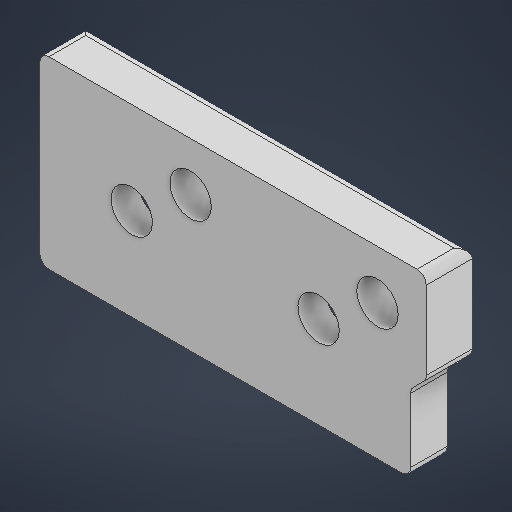
# Autodesk Inventor part: gpu_hold_plate
Saved by Autodesk Inventor 2026.2 (Build 302298010, 298A)
## iProperties
Created: 2025-02-02
Part Number: gpu_hold_plate
Material: 一般
Document SubType Name: Modeling
Designer: nyxeon
Density: 1 g/cm^3
Appearance: 既定
Author: nyxeon
Autodesk Inventor part; units mm, degrees
ref_plane "YZ Plane" through (0, 0, 0) normal (1, 0, 0) x (0, 1, 0)
ref_plane "XZ Plane" through (0, 0, 0) normal (0, 1, 0) x (-1, 0, 0)
ref_plane "XY Plane" through (0, 0, 0) normal (0, 0, 1) x (1, 0, 0)
sketch "スケッチ1" plane through (0, 0, 0) normal (0, 0, 1) x (1, 0, 0)
  arc A0 (-17.9, -5.9192) -> (-17.6, -6.2192) centre (-17.6, -5.9192) ccw construction
  line L0 (-17.6, -6.2192) -> (-11.8244, -6.2192) construction
  line L1 (-11.8244, -6.2192) -> (-9.5, -2.219) projected
  arc A1 (-9.2172, -2.0192) -> (-9.5, -2.219) centre (-9.2172, -2.3192) ccw projected
  line L2 (-9.2172, -2.0192) -> (-6.9328, -2.0192) projected
  arc A2 (-6.65, -2.219) -> (-6.9328, -2.0192) centre (-6.9328, -2.3192) ccw projected
  line L3 (-6.65, -2.219) -> (-4.3256, -6.2192) projected
  line L4 (-4.3256, -6.2192) -> (8.4756, -6.2192) construction
  line L5 (8.4756, -6.2192) -> (10.8, -2.219) projected
  arc A3 (11.0828, -2.0192) -> (10.8, -2.219) centre (11.0828, -2.3192) ccw projected
  line L6 (11.0828, -2.0192) -> (13.3672, -2.0192) projected
  arc A4 (13.65, -2.219) -> (13.3672, -2.0192) centre (13.3672, -2.3192) ccw projected
  line L7 (13.65, -2.219) -> (15.9744, -6.2192) projected
  line L8 (15.9744, -6.2192) -> (21.25, -6.2192) construction
  arc A5 (21.25, -6.2192) -> (21.55, -5.9192) centre (21.25, -5.9192) ccw construction
  line L9 (21.55, -2.3692) -> (21.55, -5.9192) construction
  arc A6 (21.55, -2.3692) -> (21.25, -2.0692) centre (21.25, -2.3692) ccw construction
  line L10 (21.25, -2.0692) -> (17.65, -2.0692) construction
  arc A7 (17.65, 2.2308) -> (17.65, -2.0692) centre (17.65, 0.0808) ccw construction
  line L11 (17.65, 2.2308) -> (21.25, 2.2308) construction
  arc A8 (21.25, 2.2308) -> (21.55, 2.5308) centre (21.25, 2.5308) ccw construction
  line L12 (21.55, 4.8808) -> (21.55, 2.5308) construction
  line L13 (21.55, 4.8808) -> (-17.9, 4.8808) construction
  line L14 (-17.9, 4.8808) -> (-17.9, -5.9192) construction
  line L15 (1.3, 1.9308) -> (1.3, -1.7692) construction
  arc A9 (1, -2.0692) -> (1.3, -1.7692) centre (1, -1.7692) ccw construction
  line L16 (1, -2.0692) -> (-2.5, -2.0692) construction
  arc A10 (-2.5, 2.2308) -> (-2.5, -2.0692) centre (-2.5, 0.0808) ccw construction
  line L17 (-2.5, 2.2308) -> (1, 2.2308) construction
  arc A11 (1.3, 1.9308) -> (1, 2.2308) centre (1, 1.9308) ccw construction
  line L18 (-17.9, 5.3808) -> (21.55, 5.3808) construction
  circle A12 centre (-0.85, 0.0808) radius 2.15 construction
  line L19 (-0.85, 0.0808) -> (-2.5, 0.0808) construction
  circle A13 centre (-1.675, 0.0808) radius 2.25
  line L20 (64.025, 2.5048) -> (64.025, 91.3712) construction
  line L21 (-65.975, 91.3712) -> (-65.975, 2.5048) construction
  line L22 (64.025, 5.3808) -> (-65.975, 5.3808)
  circle A14 centre (18.625, 0.0808) radius 2.25
  circle A15 centre (38.925, 0.0808) radius 2.25
  circle A16 centre (59.225, 0.0808) radius 2.25
  circle A17 centre (-21.975, 0.0808) radius 2.25
  circle A18 centre (-1.675, 0.0808) radius 2.25
  circle A19 centre (18.625, 0.0808) radius 2.25
  circle A20 centre (38.925, 0.0808) radius 2.25
  circle A21 centre (-42.275, 0.0808) radius 2.25
  circle A22 centre (-21.975, 0.0808) radius 2.25
  circle A23 centre (-1.675, 0.0808) radius 2.25
  circle A24 centre (18.625, 0.0808) radius 2.25
  circle A25 centre (-62.575, 0.0808) radius 2.25
  circle A26 centre (-42.275, 0.0808) radius 2.25
  circle A27 centre (-21.975, 0.0808) radius 2.25
  circle A28 centre (-1.675, 0.0808) radius 2.25
  line L23 (64.025, 5.3808) -> (64.025, -6.2192)
  line L24 (64.025, -6.2192) -> (-65.975, -6.2192)
  line L25 (-65.975, -6.2192) -> (-65.975, 5.3808)
  point P0 (0, 0)
  dimension "d1" = 4.5
  dimension "d4" = 20.3
  dimension "d7" = 20.3
  constraints: 17 centre point, 10 end point, 5 point on line, 4 horizontal, 3 tangent, 1 collinear, 1 midpoint, 1 perpendicular, 30 other
  measures "d1" diameter of A13
  measures "d4" distance of A13.centre A14.centre
  measures "d7" distance of A13.centre A17.centre
extrude "押し出し1" add sketch "スケッチ1" along normal blind 5 contours L24 L25 L22 L23 L7 A4 L6 A3 L5 L3 A2 L2 A1 L1 | L1 A1 L2 A2 L3 L24 | L5 A3 L6 A4 L7 L24 | A16 | A25
sketch "スケッチ3" plane through (0, 0, 0) normal (0, 0, -1) x (-1, 0, 0)
  line L0 (9.5, -2.219) -> (11.8244, -6.2192) projected
  arc A0 (9.5, -2.219) -> (9.2172, -2.0192) centre (9.2172, -2.3192) ccw projected
  line L1 (6.9328, -2.0192) -> (9.2172, -2.0192) projected
  arc A1 (6.9328, -2.0192) -> (6.65, -2.219) centre (6.9328, -2.3192) ccw projected
  line L2 (4.3256, -6.2192) -> (6.65, -2.219) projected
  line L3 (65.975, -6.2192) -> (-64.025, -6.2192) projected
  point P0 (0, 0)
extrude "押し出し2" cut sketch "スケッチ3" against normal through all
pattern_linear "矩形状パターン1" count 4 spacing 20.3 along (1, 0, 0) count 3 spacing 20.3 along (-1, 0, 0) of "押し出し2"
fillet "フィレット1" radius 1 1 edges at (-0.975, 5.3808, 0)
sketch "スケッチ7" plane through (0, 0, 5) normal (0, 0, 1) x (1, 0, 0)
  line L0 (-52.4244, -6.2192) -> (-50.1, -2.219) projected
  arc A0 (-49.8172, -2.0192) -> (-50.1, -2.219) centre (-49.8172, -2.3192) ccw projected
  line L1 (-49.8172, -2.0192) -> (-47.5328, -2.0192) projected
  arc A1 (-47.25, -2.219) -> (-47.5328, -2.0192) centre (-47.5328, -2.3192) ccw projected
  line L2 (-47.25, -2.219) -> (-44.9256, -6.2192) projected
  line L3 (-32.1244, -6.2192) -> (-29.8, -2.219) projected
  arc A2 (-29.5172, -2.0192) -> (-29.8, -2.219) centre (-29.5172, -2.3192) ccw projected
  line L4 (-29.5172, -2.0192) -> (-27.2328, -2.0192) projected
  arc A3 (-26.95, -2.219) -> (-27.2328, -2.0192) centre (-27.2328, -2.3192) ccw projected
  line L5 (-26.95, -2.219) -> (-24.6256, -6.2192) projected
  line L6 (-11.8244, -6.2192) -> (-9.5, -2.219) projected
  arc A4 (-9.2172, -2.0192) -> (-9.5, -2.219) centre (-9.2172, -2.3192) ccw projected
  line L7 (-9.2172, -2.0192) -> (-6.9328, -2.0192) projected
  arc A5 (-6.65, -2.219) -> (-6.9328, -2.0192) centre (-6.9328, -2.3192) ccw projected
  line L8 (-6.65, -2.219) -> (-4.3256, -6.2192) projected
  line L9 (8.4756, -6.2192) -> (10.8, -2.219) projected
  arc A6 (11.0828, -2.0192) -> (10.8, -2.219) centre (11.0828, -2.3192) ccw projected
  line L10 (11.0828, -2.0192) -> (13.3672, -2.0192) projected
  arc A7 (13.65, -2.219) -> (13.3672, -2.0192) centre (13.3672, -2.3192) ccw projected
  line L11 (13.65, -2.219) -> (15.9744, -6.2192) projected
  line L12 (28.7756, -6.2192) -> (31.1, -2.219) projected
  arc A8 (31.3828, -2.0192) -> (31.1, -2.219) centre (31.3828, -2.3192) ccw projected
  line L13 (31.3828, -2.0192) -> (33.6672, -2.0192) projected
  arc A9 (33.95, -2.219) -> (33.6672, -2.0192) centre (33.6672, -2.3192) ccw projected
  line L14 (33.95, -2.219) -> (36.2744, -6.2192) projected
  line L15 (49.0756, -6.2192) -> (51.4, -2.219) projected
  arc A10 (51.6828, -2.0192) -> (51.4, -2.219) centre (51.6828, -2.3192) ccw projected
  line L16 (51.6828, -2.0192) -> (53.9672, -2.0192) projected
  arc A11 (54.25, -2.219) -> (53.9672, -2.0192) centre (53.9672, -2.3192) ccw projected
  line L17 (54.25, -2.219) -> (56.5744, -6.2192) projected
  line L18 (-52.4244, -6.2192) -> (-44.9256, -6.2192)
  line L19 (-24.6256, -6.2192) -> (-26.95, -2.219) projected
  line L20 (-32.1244, -6.2192) -> (-24.6256, -6.2192)
  line L21 (-9.5, -2.219) -> (-11.8244, -6.2192) projected
  line L22 (-11.8244, -6.2192) -> (-4.3256, -6.2192)
  line L23 (15.9744, -6.2192) -> (8.4756, -6.2192)
  line L24 (36.2744, -6.2192) -> (33.95, -2.219) projected
  line L25 (28.7756, -6.2192) -> (36.2744, -6.2192)
  line L26 (49.0756, -6.2192) -> (56.5744, -6.2192)
  point P0 (0, 0)
  constraints: 12 end point, 4 horizontal
extrude "押し出し5" add sketch "スケッチ7" against normal blind 4
sketch "スケッチ8" plane through (0, 0, 5) normal (0, 0, 1) x (1, 0, 0)
  circle A0 centre (-42.275, 0.0808) radius 2.25 projected
  circle A1 centre (-21.975, 0.0808) radius 2.25 projected
  line L0 (-42.275, 0.0808) -> (-21.975, 0.0808) construction
  line L1 (-21.975, 0.0808) -> (-32.125, 0.0808) construction
  line L2 (-48.675, -4.6192) -> (-28.375, -4.6192) construction
  circle A2 centre (-48.675, -4.6192) radius 2.25
  circle A3 centre (-28.375, -4.6192) radius 2.25
  line L3 (-65.975, -6.2192) -> (64.025, -6.2192) projected
  line L4 (-58.675, -6.2192) -> (-18.375, -6.2192)
  line L5 (-18.375, -6.2192) -> (-18.375, -14.6192)
  line L6 (-18.375, -14.6192) -> (-58.675, -14.6192)
  line L7 (-58.675, -14.6192) -> (-58.675, -6.2192)
  line L8 (-65.975, 5.3808) -> (64.025, 5.3808) projected
  line L9 (-27.2328, -2.0192) -> (-29.5172, -2.0192) construction
  point P0 (0, 0)
  point P1 (-38.525, -14.6192)
  point P2 (-18.375, -6.2192)
  point P3 (-38.525, -4.6192)
  point P4 (-28.375, -2.0192)
  point P5 (-28.375, -2.0192)
  dimension "d43" = 20.3
  dimension "d44" = 4.5
  dimension "d45" = 10
  dimension "d46" = 10
  dimension "d53" = 6.4
  dimension "d54" = 10
  dimension "d62" = 4.5
  dimension "d63" = 20.3
  constraints: 14 end point, 5 midpoint, 3 coincident, 3 horizontal, 2 centre point, 2 parallel, 2 vertical alignment, 1 equal radius, 1 perpendicular, 1 point on line
  measures "d43" distance of L2.start L2.end
  measures "d44" diameter of A2
  measures "d45" distance from line of L6 L2.end
  measures "d46" distance from line of L2.start L7
  measures "d53" horizontal distance of point (-38.525, -4.619) L1.end
  measures "d54" distance between parallel lines of L2 L8
  measures "d62" diameter of A0
  measures "d63" distance of L0.start L0.end
extrude "押し出し6" add sketch "スケッチ8" against normal up to surface (4 mm away) contours A2 L3 A3 L5 L6 L7
sketch "スケッチ10" plane through (0, 0, 5) normal (0, 0, 1) x (1, 0, 0)
  arc A0 (-50.2569, -6.2192) -> (-47.0931, -6.2192) centre (-48.675, -4.6192) ccw construction
  arc A1 (-29.9569, -6.2192) -> (-26.7931, -6.2192) centre (-28.375, -4.6192) ccw construction
  circle A2 centre (-48.675, -4.6192) radius 2.25
  circle A3 centre (-28.375, -4.6192) radius 2.25
  point P0 (0, 0)
  constraints: 2 centre point, 2 coincident
extrude "押し出し8" cut sketch "スケッチ10" against normal through all
sketch "スケッチ11" plane through (0, 0, 1) normal (0, 0, -1) x (-1, 0, 0)
  circle A0 centre (28.375, -4.6192) radius 2.25 construction
  circle A1 centre (48.675, -4.6192) radius 2.25 construction
  circle A2 centre (28.375, -4.6192) radius 4.15
  circle A3 centre (48.675, -4.6192) radius 4.15
  point P0 (0, 0)
  dimension "d57" = 8.3
  constraints: 2 centre point, 2 coincident, 1 equal radius
  measures "d57" diameter of A2
extrude "押し出し9" cut sketch "スケッチ11" along normal blind 10 and the other way blind 1
sketch "スケッチ9" plane through (0, 0, 0) normal (0, 0, -1) x (-1, 0, 0)
  line L0 (58.675, -14.6192) -> (58.675, -6.2192) projected
  line L1 (58.675, -14.6192) -> (88.3695, -14.6192)
  line L2 (88.3695, -14.6192) -> (88.3695, 31.2927)
  line L3 (88.3695, 31.2927) -> (58.675, 31.2927)
  line L4 (58.675, 31.2927) -> (58.675, -14.6192)
  line L5 (18.375, -14.6192) -> (-64.2943, -14.6192)
  line L6 (-64.2943, -14.6192) -> (-64.2943, 35.8918)
  line L7 (-64.2943, 35.8918) -> (18.375, 35.8918)
  line L8 (18.375, 35.8918) -> (18.375, -14.6192)
  circle A0 centre (21.975, 0.0808) radius 2.25 construction
  line L9 (65.975, 5.3808) -> (-64.025, 5.3808) construction
  circle A1 centre (21.975, 0.0808) radius 5.3 construction
  line L10 (16.675, 5.3808) -> (16.675, -4.5192)
  line L11 (16.675, -4.5192) -> (18.375, -6.2192)
  line L12 (24.5458, -6.2192) -> (11.8244, -6.2192) projected
  line L13 (16.675, 5.3808) -> (18.375, 5.3808)
  point P0 (0, 0)
  dimension "d64" = 45
  constraints: 22 end point, 5 point on line, 4 parallel, 2 horizontal, 2 perpendicular, 2 tangent, 1 centre point, 1 coincident, 1 vertical
  measures "d64" angle of L8 L11
extrude "押し出し7" cut sketch "スケッチ9" against normal through all contours L0 L4 L3 L2 L1 | L5 L6 L7 L8 L13 L10 L11
fillet "フィレット2" radius 0.6 5 edges at (-32.2042, -6.2192, 0.5) (-24.5458, -6.2192, 0.5) (-52.5042, -6.2192, 0.5) (-44.8458, -6.2192, 0.5) (-58.675, -6.2192, 0.5)
fillet "フィレット2" radius 1 6 edges at (-58.675, -14.6192, 3) (-18.375, -14.6192, 3) (-58.675, 5.3808, 3) (-16.675, 5.3808, 3) (-16.675, -4.5192, 2.5) (-18.375, -6.2192, 3)
equation "\"d43\" = d63"
